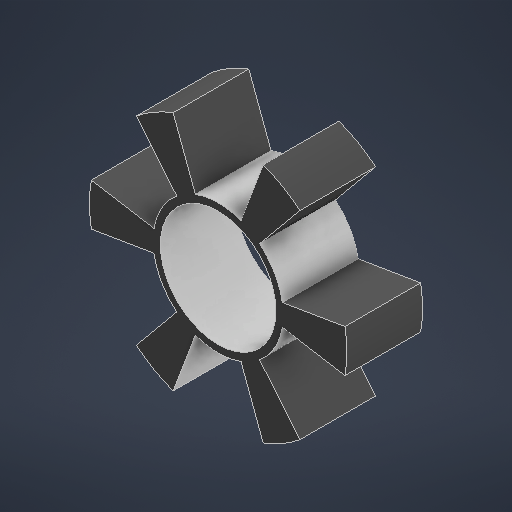
# Autodesk Inventor part: coupling_conn
Saved by Autodesk Inventor 2027 (Build 310192000, 192)
## iProperties
Category: PARTsolutions
Company: FESTO
Created: 2026-05-27
Part Number: coupling_conn
Material: Generic
Catalog Web Link: www.3dfindit.com
Description: EAMD-coupling
Vendor: FESTO
Document SubType Name: Modeling
Designer: psAdmin
Manufacturer: FESTO
Mass: 126 g
Surface Area: 117.587 cm^2
Volume: 24.6259 cm^3
Density: 1 g/cm^3
Appearance: PSOLRGB-176-176-176
PSOL_IDENT_0: {$CADENAS_DATA/23d-libs/festo/parts/e/eamd/eamd.prj},190 {VTYP=3D},{NB=558001 EAMD-32-32-11-16x20},{
PSOL_IDENT_1: LINA=558001 EAMD-32-32-11-16x20},{NN=EAMD},{DATE=05.05.2026 07:51:46},{GEOMDATE=01.09.2025 08:29:23}
PSOL_IDENT_2: ,{VERSION=},{LINEID=40},{WBVAR=},{WBNUMERIC=}  {NB=558001 EAMD-32-32-11-16x20},{LINA=558001 EAMD-32-
PSOL_IDENT_3: 32-11-16x20},{KT=DUMMY},{TNR=558001},{TYP=EAMD-32-32-11-16x20},{INFO=},{D1=11.000},{D2=16.000},{DA=0
PSOL_IDENT_4: .000},{F=0.000},{L1=0.000},{L2=0.000},{L3=0.000},{L4=0.000},{L5=0.000},{A=3.950},{VERS=3},{CNSMASSEX
PSOL_IDENT_5: ACT=0.1260},{GTIN=4052568204419},{EOLDATE=}
NB: 558001 EAMD-32-32-11-16x20
NN: EAMD
NT: coupling
NBSYN: $TNR. $TYP.
LINA: 558001 EAMD-32-32-11-16x20
CATALOG: Festo
TNR: 558001
TYP: EAMD-32-32-11-16x20
D1: 11
D2: 16
DA: 0
F: 0
L1: 0
L2: 0
L3: 0
L4: 0
L5: 0
CNSMASSEXACT: 0.126
GTIN: 4052568204419
SUPPLIER: FESTO
ARTICLENO: 558001 EAMD-32-32-11-16x20
BOMINFO: 558001 EAMD-32-32-11-16x20
CREATOR: CADENAS GmbH
Title: 558001 EAMD-32-32-11-16x20
Author: Cadenas PARTsolutions
Comments: coupling
Autodesk Inventor part; units mm, degrees
sketch "Sketch_4" plane through (0, 0, -20.7) normal (0, 0, 1) x (1, 0, 0)
  arc A0 (-15.5833, 2.6078) -> (-15.5833, -2.6078) centre (0, 0) ccw
  line L0 (-15.5833, -2.6078) -> (-7.8903, -1.3204)
  arc A1 (-7.8903, -1.3204) -> (-5.0886, -6.173) centre (0, 0) ccw
  line L1 (-5.0886, -6.173) -> (-10.05, -12.1917)
  arc A2 (-10.05, -12.1917) -> (-5.5333, -14.7994) centre (0, 0) ccw
  line L2 (-5.5333, -14.7994) -> (-2.8017, -7.4934)
  arc A3 (-2.8017, -7.4934) -> (2.8017, -7.4934) centre (0, 0) ccw
  line L3 (2.8017, -7.4934) -> (5.5333, -14.7994)
  arc A4 (5.5333, -14.7994) -> (10.05, -12.1917) centre (0, 0) ccw
  line L4 (10.05, -12.1917) -> (5.0886, -6.173)
  arc A5 (5.0886, -6.173) -> (7.8903, -1.3204) centre (0, 0) ccw
  line L5 (7.8903, -1.3204) -> (15.5833, -2.6078)
  arc A6 (15.5833, -2.6078) -> (15.5833, 2.6078) centre (0, 0) ccw
  line L6 (15.5833, 2.6078) -> (7.8903, 1.3204)
  arc A7 (7.8903, 1.3204) -> (5.0886, 6.173) centre (0, 0) ccw
  line L7 (5.0886, 6.173) -> (10.05, 12.1917)
  arc A8 (10.05, 12.1917) -> (5.5333, 14.7994) centre (0, 0) ccw
  line L8 (5.5333, 14.7994) -> (2.8017, 7.4934)
  arc A9 (2.8017, 7.4934) -> (-2.8017, 7.4934) centre (0, 0) ccw
  line L9 (-2.8017, 7.4934) -> (-5.5333, 14.7994)
  arc A10 (-5.5333, 14.7994) -> (-10.05, 12.1917) centre (0, 0) ccw
  line L10 (-10.05, 12.1917) -> (-5.0886, 6.173)
  arc A11 (-5.0886, 6.173) -> (-7.8903, 1.3204) centre (0, 0) ccw
  line L11 (-7.8903, 1.3204) -> (-15.5833, 2.6078)
  constraints: 24 end point, 24 point on circle, 12 centre point
extrude "Extrusion5" add sketch "Sketch_4" along normal blind 9.3
sketch "Sketch_9" plane through (0, 0, 0) normal (1, 0, 0) x (0, 1, 0)
  line L0 (0, -52) -> (0, 0)
  line L1 (0, 0) -> (5.5, 0)
  line L2 (5.5, 0) -> (5.5, -10.1)
  line L3 (5.5, -10.1) -> (7.1, -10.1)
  line L4 (7.1, -10.1) -> (7.1, -21.8)
  line L5 (7.1, -21.8) -> (4.5, -21.8)
  line L6 (4.5, -21.8) -> (4.5, -24.3)
  line L7 (4.5, -24.3) -> (2.067, -24.3)
  line L8 (2.067, -24.3) -> (2.067, -51.567)
  line L9 (2.067, -51.567) -> (2.5, -52)
  line L10 (2.5, -52) -> (0, -52)
  line L11 (0, -52) -> (0, 0)
  constraints: 24 end point
revolve "Revolution3" cut sketch "Sketch_9" angle 360 about axis through (0, 0, -52) along (0, 0, -1)
ref_plane "KUPPLUNG_XY" through (0, 0, 0) normal (0, 0, 1) x (1, 0, 0)
ref_plane "KUPPLUNG_YZ" through (0, 0, 0) normal (1, 0, 0) x (0, 1, 0)
ref_plane "KUPPLUNG_ZX" through (0, 0, 0) normal (0, 1, 0) x (0, 0, 1)
body "Solid1"
